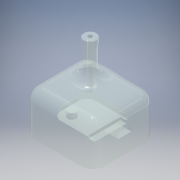
# Autodesk Inventor part: DAQcapsule
Saved by Autodesk Inventor 2018 (Build 220112000, 112)
## iProperties
Created: 2020-03-04
Part Number: DAQcapsule
Material: Generic
Document SubType Name: Modeling
Designer: Ivan
Density: 1 g/cm^3
Appearance: Default
Author: Ivan
Autodesk Inventor part; units mm, degrees
ref_plane "YZ Plane" through (0, 0, 0) normal (1, 0, 0) x (0, 1, 0)
ref_plane "XY Plane" through (0, 0, 0) normal (0, 0, 1) x (1, 0, 0)
sketch "Sketch1" plane through (0, 0, 0) normal (0, 0, 1) x (1, 0, 0)
  line L0 (0, 0) -> (24, 0)
  line L1 (24, 0) -> (24, 22)
  line L2 (24, 22) -> (0, 22)
  line L3 (0, 22) -> (0, 0)
  dimension "d0" = 24
  dimension "d1" = 22
  constraints: 8 end point, 2 parallel, 1 horizontal, 1 perpendicular
  measures "d0" distance of L2.end L1.end
  measures "d1" distance of L1.end L0.end
extrude "Extrusion1" add sketch "Sketch1" along normal blind 5
sketch "Sketch2" plane through (0, 0, 5) normal (0, 0, 1) x (1, 0, 0)
  circle A0 centre (8.5, 8.25) radius 1.45
  line L0 (0, 0) -> (24, 0) projected
  line L1 (0, 22) -> (0, 0) projected
  dimension "d6" = 2.9
  dimension "d7" = 8.25
  dimension "d8" = 8.5
  constraints: 1 centre point
  measures "d6" diameter of A0
  measures "d7" distance from line of L0 A0.centre
  measures "d8" distance from line of L1 A0.centre
extrude "Extrusion2" add sketch "Sketch2" along normal blind 2
sketch "Sketch3" plane through (0, 0, 5) normal (0, 0, 1) x (1, 0, 0)
  line L0 (17, 5.5) -> (19, 5.5)
  line L1 (19, 5.5) -> (19, 16.5)
  line L2 (19, 16.5) -> (17, 16.5)
  line L3 (17, 16.5) -> (17, 5.5)
  line L4 (0, 0) -> (24, 0) projected
  line L5 (0, 22) -> (0, 0) projected
  circle A0 centre (8.5, 8.25) radius 1.45 construction
  dimension "d9" = 2
  dimension "d10" = 11
  dimension "d58" = 8.5
  dimension "d59" = 2.75
  constraints: 8 end point, 2 parallel, 1 horizontal, 1 perpendicular
  measures "d9" distance of L2.end L1.end
  measures "d10" distance of L1.end L0.end
  measures "d58" distance from line of L3 A0.centre
  measures "d59" distance from line of A0.centre L0
extrude "Extrusion3" cut sketch "Sketch3" against normal blind 1
sketch "Sketch4" plane through (0, 0, 5) normal (0, 0, 1) x (1, 0, 0)
  line L0 (0, 22) -> (24, 22)
  line L1 (24, 22) -> (24, 17)
  line L2 (24, 17) -> (0, 17)
  line L3 (0, 17) -> (0, 22)
  line L4 (24, 0) -> (24, 22) construction
  line L5 (24, 17) -> (19, 17)
  line L6 (19, 17) -> (19, 0)
  line L7 (19, 0) -> (24, 0)
  line L8 (24, 0) -> (24, 17)
  line L9 (0, 0) -> (24, 0) projected
  line L10 (19, 0) -> (0, 0)
  line L11 (0, 0) -> (0, 5)
  line L12 (0, 5) -> (19, 5)
  line L13 (19, 5) -> (19, 0)
  line L14 (0, 22) -> (0, 0) projected
  line L15 (0, 5) -> (5, 5)
  line L16 (5, 5) -> (5, 17)
  line L17 (5, 17) -> (0, 17)
  line L18 (0, 17) -> (0, 5)
  dimension "d16" = 5
  dimension "d17" = 5
  dimension "d18" = 5
  dimension "d19" = 5
  constraints: 32 end point, 8 parallel, 4 collinear, 4 horizontal, 4 perpendicular
  measures "d16" distance of L0.end L1.end
  measures "d17" distance between parallel lines of L4 L6
  measures "d18" distance between parallel lines of L12 L9
  measures "d19" distance between parallel lines of L16 L18
extrude "Extrusion4" add sketch "Sketch4" along normal blind 4 contours L0 L1 L2 L3 | L2 L16 L12 L14 | L8 L7 L6 L2 | L12 L6 L9 L11
ref_plane "Work Plane2" through (0, 11, 0) normal (0, 1, 0) x (-1, 0, 0)
sketch "Sketch15" plane through (0, 0, 9) normal (0, 0, 1) x (1, 0, 0)
  line L0 (24, 22) -> (0, 22) projected
  line L1 (0, 22) -> (0, 0) projected
  line L2 (0, 0) -> (24, 0) projected
  line L3 (24, 0) -> (24, 22) projected
extrude "Extrusion15" add sketch "Sketch15" along normal blind 5
sketch "Sketch18" plane through (0, 0, 14) normal (0, 0, 1) x (1, 0, 0)
  circle A0 centre (9.25, 13.75) radius 2
  circle A1 centre (8.5, 8.25) radius 1.45 construction
  point P0 (0, 0)
  dimension "d70" = 4
  dimension "d107" = 5.5
  dimension "d108" = 0.75
  constraints: 1 centre point
  measures "d70" diameter of A0
  measures "d107" vertical distance of A0.centre A1.centre
  measures "d108" horizontal distance of A0.centre A1.centre
extrude "Extrusion17" add sketch "Sketch18" along normal blind 10
fillet "Fillet5" radius 4 1 edges at (7.25, 13.75, 14)
fillet "Fillet6" radius 4 8 edges at (0, 11, 14) (12, 0, 14) (24, 11, 14) (12, 22, 14) (0, 0, 7) (24, 0, 7) (0, 22, 7) (24, 22, 7)
ref_plane "Work Plane4" through (9.25, 13.75, 26.5) normal (0, 0, 1) x (1, 0, 0)
sketch "Sketch21" plane through (9.25, 13.75, 26.5) normal (0, 0, 1) x (1, 0, 0)
  circle A0 centre (0, 0) radius 2 construction
  circle A1 centre (0, 0) radius 2.25
  point P0 (-9.25, -13.75)
  dimension "d91" = 0.25
  constraints: 1 centre point, 1 coincident
  measures "d91" radial gap between concentric circles of A0 A1
loft "Loft3" add profiles "Sketch21" section 2 edges at (7.25, 13.75, 24)
fillet "Fillet8" radius 0.25 1 edges at (7, 13.75, 26.5)
fillet "Fillet9" radius 2 1 edges at (7.25, 13.75, 24)
sketch "Sketch22" plane through (9.25, 13.75, 26.5) normal (0, 0, 1) x (1, 0, 0)
  circle A0 centre (0, 0) radius 0.75
  point P0 (-9.25, -13.75)
  dimension "d98" = 1.5
  constraints: 1 centre point
  measures "d98" diameter of A0
extrude "Extrusion19" cut sketch "Sketch22" against normal blind 20
sketch "Sketch23" plane through (24, 4, 0) normal (1, 0, 0) x (0, 0, -1)
  line L0 (-9, 13) -> (-9, 1) construction
  line L1 (-5.75, 4.75) -> (-5.75, 9.25)
  line L2 (-7.5, 4.75) -> (-7.5, 9.25)
  line L3 (-5.75, 4.75) -> (-7.5, 4.75)
  line L4 (-5, 1.5) -> (-5, 12.5) projected
  line L5 (-7.5, 9.25) -> (-5.75, 9.25)
  point P0 (0, -4)
  point P1 (-9, 7)
  point P2 (-9, 7)
  dimension "d104" = 4.5
  dimension "d111" = 1.5
  dimension "d112" = 1.75
  constraints: 8 end point, 1 coincident, 1 midpoint, 1 parallel, 1 perpendicular
  measures "d104" distance of L1.end L1.start
  measures "d111" distance from line of point (-9, 7) L2
  measures "d112" distance of L2.end L1.end
extrude "Extrusion20" cut sketch "Sketch23" against normal blind 5
fillet "Fillet10" radius 3.5 2 edges at (12, 17, 9) (12, 5, 9)
fillet "Fillet11" radius 3 5 edges at (5, 15.9749, 7.9749) (5, 17, 5.25) (5, 6.0251, 7.9749) (5, 5, 5.25) (5, 11, 9)
equation "\"d17\" = d16"
equation "\"d18\" = d16"
equation "\"d19\" = d16"
body "Solid1"
